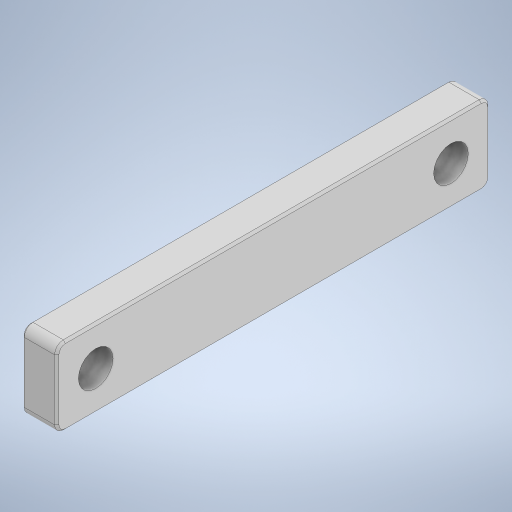
# Autodesk Inventor part: HUDSON 1-03 AXLE BOX KEEPER
Saved by Autodesk Inventor 2024.2 (Build 282272000, 272)
## iProperties
Created: 2024-09-30
Part Number: HUDSON 1-03 AXLE BOX KEEPER
Material: Generic
Document SubType Name: Modeling
Designer: Jimena Brenes
Density: 1 g/cm^3
Appearance: Default
Author: Jimena Brenes
Autodesk Inventor part; units mm, degrees
ref_plane "YZ Plane" through (0, 0, 0) normal (1, 0, 0) x (0, 1, 0)
ref_plane "XZ Plane" through (0, 0, 0) normal (0, 1, 0) x (-1, 0, 0)
ref_plane "XY Plane" through (0, 0, 0) normal (0, 0, 1) x (1, 0, 0)
sketch "Sketch1" plane through (0, 0, 0) normal (0, 0, 1) x (1, 0, 0)
  line L0 (0, 0) -> (4, 0)
  line L1 (4, 0) -> (4, 9)
  line L2 (4, 9) -> (0, 9)
  line L3 (0, 9) -> (0, 0)
  dimension "d3" = 4
  dimension "d4" = 9
  constraints: 8 end point, 2 parallel, 1 horizontal, 1 perpendicular
  measures "d3" distance between parallel lines of L1 L3
  measures "d4" distance between parallel lines of L2 L0
extrude "Extrusion1" add sketch "Sketch1" against normal blind 50
sketch "Sketch2" plane through (4, 0, 0) normal (1, 0, 0) x (0, 0, -1)
  circle A0 centre (4.5, 4.5) radius 2
  circle A1 centre (45.5, 4.5) radius 2
  line L0 (0, 0) -> (50, 0) projected
  line L1 (0, 0) -> (0, 9) projected
  line L2 (50, 9) -> (50, 0) projected
  line L3 (0, 9) -> (50, 9) projected
  dimension "d7" = 4
  dimension "d8" = 4
  dimension "d9" = 4.5
  dimension "d10" = 4.5
  dimension "d11" = 41
  dimension "d12" = 4.5
  dimension "d13" = 4.5
  constraints: 2 centre point
  measures "d7" diameter of A0
  measures "d8" diameter of A1
  measures "d9" distance from line of L0 A0.centre
  measures "d10" distance from line of L1 A0.centre
  measures "d11" distance of A1.centre A0.centre
  measures "d12" distance from line of L2 A1.centre
  measures "d13" distance from line of L3 A1.centre
hole "Hole1" at (4, 4.5, -4.5) at (4, 4.5, -45.5) direction (-1, 0, 0) diameter 4 depth 4 tip angle 118
fillet "Fillet1" radius 1 4 edges at (2, 9, 0) (2, 0, 0) (2, 9, -50) (2, 0, -50)
chamfer "Chamfer1" distance 0.25 angle 45 16 edges at (0, 9, -25) (0, 8.7071, -49.7071) (0, 4.5, -50) (0, 0.2929, -49.7071) (0, 0, -25) (0, 0.2929, -0.2929) (0, 4.5, 0) (0, 8.7071, -0.2929) (4, 0, -25) (4, 0.2929, -49.7071) (4, 4.5, -50) (4, 8.7071, -49.7071) (4, 9, -25) (4, 8.7071, -0.2929) (4, 4.5, 0) (4, 0.2929, -0.2929)
body "Solid1"
